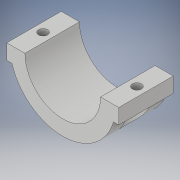
# Autodesk Inventor part: Clamp_Mount
Saved by Autodesk Inventor 2019 (Build 230136000, 136)
## iProperties
Created: 2019-10-22
Part Number: Clamp_Mount
Material: Generic
Document SubType Name: Modeling
Designer: 19879326
Density: 1 g/cm^3
Appearance: Default
Author: 19879326
Autodesk Inventor part; units mm, degrees
ref_plane "YZ Plane" through (0, 0, 0) normal (1, 0, 0) x (0, 1, 0)
ref_plane "XZ Plane" through (0, 0, 0) normal (0, 1, 0) x (-1, 0, 0)
ref_plane "XY Plane" through (0, 0, 0) normal (0, 0, 1) x (1, 0, 0)
sketch "Sketch1" plane through (0, 0, 0) normal (0, 0, 1) x (1, 0, 0)
  arc A0 (-12.5, 0) -> (12.5, 0) centre (0, 0) ccw
  arc A1 (-16.7705, -5) -> (16.7705, -5) centre (0, 0) ccw
  line L0 (-16.5, 0) -> (-18.5, 0)
  line L1 (-18.5, 0) -> (-18.5, -5)
  line L2 (-18.5, -5) -> (-16.7705, -5)
  line L3 (16.5, 0) -> (18.5, 0)
  line L4 (18.5, 0) -> (18.5, -5)
  line L5 (18.5, -5) -> (16.7705, -5)
  line L6 (-16.5, 0) -> (-12.5, 0)
  line L7 (12.5, 0) -> (16.5, 0)
  point P0 (-17.5, 0)
  dimension "d0" = 25
  dimension "d2" = 5
  dimension "d3" = 2
  dimension "d4" = 5
  dimension "d22" = 6
  constraints: 16 end point, 5 point on line, 4 point on circle, 3 collinear, 3 perpendicular, 2 centre point, 2 coincident, 2 horizontal, 1 horizontal alignment, 1 midpoint
  measures "d0" diameter of A0
  measures "d2" radial gap between concentric circles of A1 A0
  measures "d3" distance of L0.start L0.end
  measures "d4" distance of L3.end L4.end
  measures "d22" distance from line of L1 L6.end
extrude "Extrusion1" add sketch "Sketch1" along normal blind 18
sketch "Sketch2" plane through (-18.5, 0, 0) normal (0, 1, 0) x (1, 0, 0)
  circle A0 centre (3, -9) radius 1.5
  circle A1 centre (34, -9) radius 1.5
  line L0 (6, 0) -> (0, 0) projected
  line L1 (37, 0) -> (31, 0) projected
  line L2 (37, 0) -> (37, -18) projected
  line L3 (0, 0) -> (0, -18) projected
  line L4 (6, 0) -> (6, -18) projected
  line L5 (31, 0) -> (31, -18) projected
  point P0 (18.5, 0)
  dimension "d8" = 3
  dimension "d9" = 3
  dimension "d10" = 9
  dimension "d11" = 9
  dimension "d16" = 3
  dimension "d17" = 3
  constraints: 2 centre point
  measures "d8" diameter of A0
  measures "d9" diameter of A1
  measures "d10" distance from line of L0 A0.centre
  measures "d11" distance from line of L1 A1.centre
  measures "d16" distance from line of L4 A0.centre
  measures "d17" distance from line of A1.centre L5
extrude "Extrusion2" cut sketch "Sketch2" against normal blind 18
sketch "Sketch3" plane through (-18.5, -5, 0) normal (0, -1, 0) x (1, 0, 0)
  circle A0 centre (3, 9) radius 1.5 projected
  circle A1 centre (3, 9) radius 4
  circle A2 centre (34, 9) radius 1.5 projected
  circle A3 centre (34, 9) radius 4
  point P0 (18.5, 0)
  dimension "d18" = 8
  dimension "d19" = 8
  constraints: 2 centre point, 2 coincident
  measures "d18" diameter of A1
  measures "d19" diameter of A3
extrude "Extrusion3" cut sketch "Sketch3" along normal blind 10
body "Solid1"
